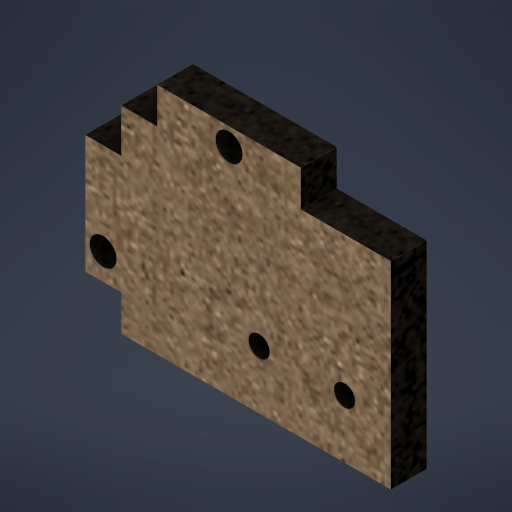
# Autodesk Inventor part: Door_LimitSwitch_Holder_Plate
Saved by Autodesk Inventor 2024.1 (Build 281209000, 209)
## iProperties
Created: 2023-08-06
Part Number: Door_LimitSwitch_Holder_Plate
Material: MDF Medium Density Fiberboard
Document SubType Name: Modeling
Designer: jaege
Density: 0.8 g/cm^3
Appearance: Cardboard - Corrugated
Author: jaege
Autodesk Inventor part; units mm, degrees
ref_plane "YZ Plane" through (0, 0, 0) normal (1, 0, 0) x (0, 1, 0)
ref_plane "XZ Plane" through (0, 0, 0) normal (0, 1, 0) x (-1, 0, 0)
ref_plane "XY Plane" through (0, 0, 0) normal (0, 0, 1) x (1, 0, 0)
sketch "Sketch1" plane through (0, 0, 0) normal (0, 0, 1) x (1, 0, 0)
  line L0 (16, 0) -> (16, 4) projected
  line L1 (0, 0) -> (0, 4) projected
  line L2 (-4, -4.8304) -> (-8, -4.8304) projected
  line L3 (-4, -18) -> (-8, -18) projected
  line L4 (-4, -4.8304) -> (-4, 0)
  line L5 (-4, 0) -> (0, 0)
  line L6 (0, 4) -> (16, 4)
  line L7 (-8, -4.8304) -> (-8, -18)
  line L8 (-4, -22) -> (-4, -18)
  line L9 (16, 0) -> (26, 0)
  line L10 (-4, -22) -> (26, -22)
  line L11 (26, -22) -> (26, 0)
  line L12 (6.5, 0) -> (6.5, 4) construction
  line L13 (9.5, 0) -> (9.5, 4) construction
  line L14 (-4, -13.56) -> (-8, -13.56) construction
  line L15 (-4, -16.56) -> (-8, -16.56) construction
  line L16 (-8, -16.56) -> (-4, -13.56) construction
  line L17 (6.5, 0) -> (9.5, 4) construction
  circle A0 centre (8, 2) radius 1.5
  circle A1 centre (-6, -15.06) radius 1.5
  circle A2 centre (11.35, -15.5) radius 1.175
  circle A3 centre (20.85, -15.5) radius 1.175
  dimension "d0" = 3
  dimension "d3" = 2.35
  dimension "d4" = 9.5
  dimension "d5" = 6.5
  dimension "d6" = 5.15
  constraints: 20 end point, 4 centre point, 4 perpendicular, 2 equal radius, 2 horizontal, 2 midpoint, 1 horizontal alignment, 1 parallel, 1 vertical, 2 other
  measures "d0" diameter of A0
  measures "d3" diameter of A3
  measures "d4" distance of A3.centre A2.centre
  measures "d5" distance from line of L10 A3.centre
  measures "d6" distance from line of A3.centre L11
extrude "Extrusion1" add sketch "Sketch1" along normal blind 4
body "Solid1"
